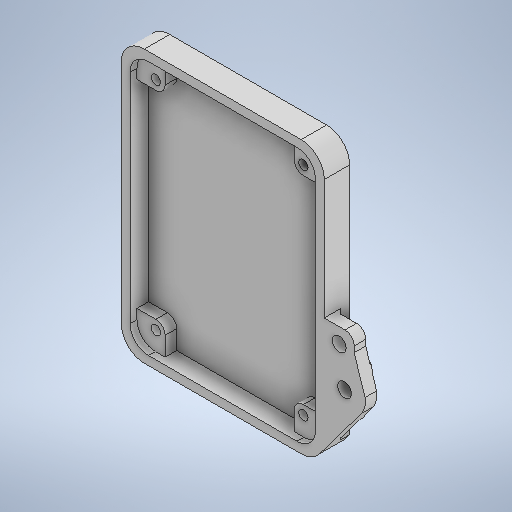
# Autodesk Inventor part: RPi_PD_Trigger
Saved by Autodesk Inventor 2025.1 (Build 291241000, 241)
## iProperties
Created: 2026-04-13
Part Number: RPi_PD_Trigger
Material: Generic
Document SubType Name: Modeling
Designer: User
Density: 1 g/cm^3
Appearance: Default
Author: User
## iProperties of the stored document RPi_PD_Trigger_3DPrint.ipt
Created: 2026-05-05
Part Number: RPi_PD_Trigger_3DPrint
Material: Generic
Document SubType Name: Modeling
Designer: User
Density: 1 g/cm^3
Appearance: Default
Author: User
Autodesk Inventor part; units mm, degrees
ref_plane "YZ Plane" through (0, 0, 0) normal (1, 0, 0) x (0, 1, 0)
ref_plane "XZ Plane" through (0, 0, 0) normal (0, 1, 0) x (-1, 0, 0)
ref_plane "XY Plane" through (0, 0, 0) normal (0, 0, 1) x (1, 0, 0)
sketch "Sketch1" plane through (0, 0, 0) normal (0, 0, 1) x (1, 0, 0)
  line L0 (8.0175, 59.5034) -> (-31.9825, 59.5034)
  line L1 (-31.9825, 59.5034) -> (-31.9825, 4.5034)
  line L2 (-31.9825, 4.5034) -> (8.0175, 4.5034)
  line L3 (8.0175, 4.5034) -> (8.0175, 59.5034)
  line L4 (10.0175, 61.5034) -> (-33.9825, 61.5034)
  line L5 (-33.9825, 61.5034) -> (-33.9825, 2.5034)
  line L6 (-33.9825, 2.5034) -> (10.0175, 2.5034)
  line L7 (10.0175, 2.5034) -> (10.0175, 61.5034)
  line L8 (-32.0825, 4.4034) -> (-32.0825, 59.6034)
  line L9 (-32.0825, 59.6034) -> (8.1175, 59.6034)
  line L10 (8.1175, 59.6034) -> (8.1175, 4.4034)
  line L11 (8.1175, 4.4034) -> (-32.0825, 4.4034)
  point P0 (0, 0)
  dimension "d0" = 40
  dimension "d1" = 55
  dimension "d17" = 2
  dimension "d18" = 59
  dimension "d19" = 44
  dimension "d20" = 0.1
  constraints: 24 end point, 6 parallel, 3 perpendicular, 1 horizontal, 6 other
  measures "d0" distance of L2.end L1.end
  measures "d1" distance of L1.end L0.end
  measures "d17" distance between parallel lines of L3 L7
  measures "d18" distance of L4.end L5.end
  measures "d19" distance of L5.end L6.end
  measures "d20" distance between parallel lines of L1 L8
extrude "Extrusion1" add sketch "Sketch1" along normal blind 5.5 contours L7 L6 L5 L4
sketch "Sketch2" plane through (0, 0, 5.5) normal (0, 0, 1) x (1, 0, 0)
  line L0 (-31.9814, 4.5065) -> (-31.9814, 59.8269) construction
  line L1 (-31.9814, 59.8269) -> (7.0141, 59.8269) construction
  line L2 (7.0141, 59.8269) -> (7.0141, 4.5065) construction
  line L3 (7.0141, 4.5065) -> (-31.9814, 4.5065) construction
  point P0 (0, 0)
  constraints: 2 other
sketch "Sketch5" plane through (0, 0, 0) normal (0, 0, -1) x (-1, 0, 0)
  line L0 (-8.1175, 4.4034) -> (32.0825, 4.4034) projected
  line L1 (-8.1175, 59.6034) -> (-8.1175, 4.4034) projected
  line L2 (32.0825, 4.4034) -> (32.0825, 59.6034) projected
  line L3 (32.0825, 59.6034) -> (-8.1175, 59.6034) projected
  point P0 (0, 0)
extrude "Extrusion4" add sketch "Sketch5" against normal blind 1.5
sketch "Sketch6" plane through (0, 0, 1.5) normal (0, 0, 1) x (1, 0, 0)
  line L0 (10.0175, 61.5034) -> (-33.9825, 61.5034) projected
  line L1 (-33.9825, 61.5034) -> (-33.9825, 2.5034) projected
  line L2 (-33.9825, 2.5034) -> (10.0175, 2.5034) projected
  line L3 (10.0175, 2.5034) -> (10.0175, 61.5034) projected
  line L4 (-33.9825, 61.5034) -> (-25.9825, 61.5034)
  line L5 (-25.9825, 61.5034) -> (-25.9825, 55.5034)
  line L6 (-27.9825, 53.5034) -> (-33.9825, 53.5034)
  line L7 (-33.9825, 53.5034) -> (-33.9825, 61.5034)
  line L8 (10.0175, 61.5034) -> (2.0175, 61.5034)
  line L9 (2.0175, 61.5034) -> (2.0175, 55.5034)
  line L10 (4.0175, 53.5034) -> (10.0175, 53.5034)
  line L11 (10.0175, 53.5034) -> (10.0175, 61.5034)
  line L12 (10.0175, 2.5034) -> (10.0175, 61.5034) projected
  line L13 (10.0175, 2.5034) -> (2.0175, 2.5034)
  line L14 (2.0175, 2.5034) -> (2.0175, 8.5034)
  line L15 (4.0175, 10.5034) -> (10.0175, 10.5034)
  line L16 (10.0175, 10.5034) -> (10.0175, 2.5034)
  line L17 (-33.9825, 2.5034) -> (10.0175, 2.5034) projected
  line L18 (-33.9825, 2.5034) -> (-25.9825, 2.5034)
  line L19 (-25.9825, 2.5034) -> (-25.9825, 8.5034)
  line L20 (-27.9825, 10.5034) -> (-33.9825, 10.5034)
  line L21 (-33.9825, 10.5034) -> (-33.9825, 2.5034)
  arc A0 (-25.9825, 8.5034) -> (-27.9825, 10.5034) centre (-27.9825, 8.5034) ccw
  arc A1 (4.0175, 10.5034) -> (2.0175, 8.5034) centre (4.0175, 8.5034) ccw
  arc A2 (2.0175, 55.5034) -> (4.0175, 53.5034) centre (4.0175, 55.5034) ccw
  arc A3 (-27.9825, 53.5034) -> (-25.9825, 55.5034) centre (-27.9825, 55.5034) ccw
  circle A4 centre (-27.9825, 55.5034) radius 1
  circle A5 centre (4.0175, 55.5034) radius 1
  circle A6 centre (-27.9825, 8.5034) radius 1
  circle A7 centre (4.0175, 8.5034) radius 1
  point P0 (0, 0)
  point P1 (-25.9825, 53.5034)
  point P2 (2.0175, 53.5034)
  point P3 (2.0175, 10.5034)
  point P4 (-25.9825, 10.5034)
  dimension "d24" = 8
  dimension "d25" = 8
  dimension "d26" = 8
  dimension "d27" = 8
  dimension "d28" = 8
  dimension "d29" = 8
  dimension "d30" = 8
  dimension "d31" = 8
  dimension "d32" = 2
  dimension "d33" = 2
  dimension "d34" = 2
  dimension "d35" = 2
  dimension "d36" = 2
  constraints: 32 end point, 8 centre point, 8 parallel, 8 point on circle, 8 point on line, 8 tangent, 4 coincident, 4 horizontal, 4 perpendicular, 3 equal radius
  measures "d24" distance of point (-25.983, 53.503) L6.end
  measures "d25" distance of L4.end point (-25.983, 53.503)
  measures "d26" distance of L10.end point (2.017, 53.503)
  measures "d27" distance of point (2.017, 53.503) L8.end
  measures "d28" distance of point (2.017, 10.503) L15.end
  measures "d29" distance of L13.end point (2.017, 10.503)
  measures "d30" distance of L20.end point (-25.983, 10.503)
  measures "d31" distance of point (-25.983, 10.503) L18.end
  measures "d32" radius of A0
  measures "d33" diameter of A4
  measures "d34" diameter of A5
  measures "d35" diameter of A6
  measures "d36" diameter of A7
extrude "Extrusion5" add sketch "Sketch6" along normal blind 2.5 contours L3 L10 A2 L9 L0 | L5 A3 L6 L1 L0 | L3 L2 L14 A1 L15 | L20 A0 L19 L2 L1
fillet "Fillet2" radius 4 4 edges at (-32.0825, 4.4034, 4.75) (-32.0825, 59.6034, 4.75) (8.1175, 59.6034, 4.75) (8.1175, 4.4034, 4.75)
fillet "Fillet3" radius 5 4 edges at (10.0175, 2.5034, 2.75) (10.0175, 61.5034, 2.75) (-33.9825, 61.5034, 2.75) (-33.9825, 2.5034, 2.75)
sketch "Sketch7" plane through (0, 0, 5.5) normal (0, 0, 1) x (1, 0, 0)
  line L0 (10.0175, 7.5034) -> (10.0175, 56.5034) projected
  line L1 (-28.9825, 2.5034) -> (5.0175, 2.5034) projected
  line L2 (5.0175, 2.5034) -> (5.0175, 30.5034)
  line L3 (10.0175, 30.5034) -> (14.5175, 30.5034)
  line L4 (16.5175, 28.5034) -> (16.5175, 4.5034)
  line L5 (10.0175, 2.5034) -> (10.0175, 30.5034)
  arc A0 (5.0175, 2.5034) -> (10.0175, 7.5034) centre (5.0175, 7.5034) ccw projected
  line L6 (5.0175, 2.5034) -> (14.5175, 2.5034)
  arc A1 (5.0175, 2.5034) -> (10.0175, 7.5034) centre (5.0175, 7.5034) ccw projected
  arc A2 (16.5175, 28.5034) -> (14.5175, 30.5034) centre (14.5175, 28.5034) ccw
  arc A3 (14.5175, 2.5034) -> (16.5175, 4.5034) centre (14.5175, 4.5034) ccw
  line L7 (10.0175, 30.5034) -> (16.5175, 30.5034)
  line L8 (16.5175, 30.5034) -> (16.5175, 24.0034)
  line L9 (16.5175, 24.0034) -> (10.0175, 24.0034)
  line L10 (10.0175, 24.0034) -> (10.0175, 30.5034)
  line L11 (16.5175, 24.0034) -> (10.0175, 30.5034)
  circle A4 centre (13.2675, 27.2534) radius 1.5
  point P0 (0, 0)
  point P1 (16.5175, 2.5034)
  dimension "d42" = 28
  dimension "d44" = 6.5
  dimension "d45" = 2
  dimension "d46" = 2
  dimension "d47" = 6.5
  dimension "d48" = 3
  constraints: 20 end point, 5 tangent, 4 point on circle, 4 point on line, 3 centre point, 3 parallel, 2 horizontal, 2 perpendicular, 1 midpoint, 1 vertical
  measures "d42" distance of L1.end L2.end
  measures "d44" distance of point (16.517, 2.503) L5.start
  measures "d45" radius of A2
  measures "d46" radius of A3
  measures "d47" distance of L7.end L8.end
  measures "d48" diameter of A4
extrude "Extrusion6" add sketch "Sketch7" against normal up to surface (5.5 mm away) contours L0 L9 L4 A3 L6 L5 | L5 L6 A0 | L0 L11 A4 L9 | L3 A2 L4 L11 A4
sketch "Sketch8" plane through (0, 0, 5.5) normal (0, 0, 1) x (1, 0, 0)
  circle A0 centre (14.4423, 19.236) radius 1.5 projected
  point P0 (0, 0)
extrude "Extrusion7" cut sketch "Sketch8" against normal blind 10
sketch "Sketch9" plane through (0, 0, 5.5) normal (0, 0, 1) x (1, 0, 0)
  circle A0 centre (14.4423, 19.236) radius 1.5 projected
  circle A1 centre (14.4423, 19.236) radius 4.5
  line L0 (16.5175, 4.5034) -> (16.5175, 28.5034) projected
  point P0 (0, 0)
  point P1 (16.5175, 23.229)
  point P2 (16.5175, 15.2431)
  dimension "d53" = 3
  constraints: 1 centre point
  measures "d53" radial gap between concentric circles of A0 A1
extrude "Extrusion8" add sketch "Sketch9" against normal up to surface (5.5 mm away) contours A1 L0 picked at (17.8338, 18.9111)
sketch "Sketch10" plane through (0, 0, 5.5) normal (0, 0, 1) x (1, 0, 0)
  line L0 (10.0175, 30.5034) -> (10.0175, 56.5034) projected
  line L1 (-28.9825, 2.5034) -> (14.5175, 2.5034) projected
  line L2 (8.1175, 55.6034) -> (8.1175, 8.4034) projected
  line L3 (4.1175, 4.4034) -> (-28.0825, 4.4034) projected
  line L4 (10.0175, 34.9354) -> (10.0175, 2.5034)
  line L5 (16.5175, 4.5034) -> (16.5175, 15.2431) projected
  line L6 (0, 4.4034) -> (16.5175, 4.5034)
  circle A0 centre (5.0175, 7.5034) radius 5
  arc A1 (16.5175, 15.2431) -> (16.5175, 23.229) centre (14.4423, 19.236) ccw projected
  line L7 (4.2612, -1.838) -> (20.9867, 20.4617)
  arc A2 (14.5175, 2.5034) -> (16.5175, 4.5034) centre (14.5175, 4.5034) ccw projected
  point P0 (0, 0)
  point P1 (16.5175, 14.503)
  point P2 (8.9832, 4.4578)
  point P3 (8.9828, 4.4578)
  point P4 (5.0175, 2.5034)
  dimension "d56" = 10
  constraints: 6 end point, 4 point on line, 4 tangent, 1 centre point
  measures "d56" diameter of A0
extrude "Extrusion9" cut sketch "Sketch10" against normal blind 10 contours L4 L6 A2 L1 | L1 L7 L6 L4 | L1 A0 L7 | L6 L7 L4 | L4 L7 L5 L6
sketch "Sketch11" plane through (0, 0, 5.5) normal (0, 0, 1) x (1, 0, 0)
  arc A0 (16.5175, 15.2431) -> (16.5175, 23.229) centre (14.4423, 19.236) ccw projected
  line L0 (8.9832, 4.4578) -> (16.5175, 14.503) projected
  line L1 (14.193, 11.4039) -> (18.0422, 16.536)
  line L2 (16.5175, 14.503) -> (16.5175, 15.2431) projected
  point P0 (0, 0)
  constraints: 2 end point, 2 point on line, 1 point on circle
extrude "Extrusion10" add sketch "Sketch11" against normal up to surface (5.5 mm away)
chamfer "Chamfer1" distance 4 angle 45 1 edges at (16.5175, 23.229, 2.75)
sketch "Sketch12" plane through (0, 0, 0) normal (0, 0, -1) x (-1, 0, 0)
  line L0 (-10.0175, 30.5034) -> (-10.0175, 56.5034) projected
  line L1 (-10.0175, 30.5034) -> (-14.5175, 30.5034) projected
  arc A0 (-14.5175, 30.5034) -> (-16.5175, 28.5034) centre (-14.5175, 28.5034) ccw projected
  line L2 (-16.5175, 28.5034) -> (-16.5175, 27.229) projected
  line L3 (-18.8771, 19.9991) -> (-16.5175, 27.229) projected
  arc A1 (-18.8771, 19.9991) -> (-18.0422, 16.536) centre (-14.4423, 19.236) ccw projected
  line L4 (-18.0422, 16.536) -> (-8.9832, 4.4578) projected
  arc A2 (-8.9828, 4.4578) -> (-5.0175, 2.5034) centre (-5.0175, 7.5034) ccw projected
  line L5 (-10.0175, 38.8161) -> (-10.0175, 5.8367)
  point P0 (0, 0)
  constraints: 3 point on line, 2 end point
extrude "Extrusion11" cut sketch "Sketch12" against normal blind 3
chamfer "Chamfer2" distance 1 angle 45 1 edges at (10.0175, 18.1701, 3)
sketch "Sketch13" plane through (0, 0, 0) normal (0, 0, -1) x (-1, 0, 0)
  line L0 (-10.0175, 5.8367) -> (-10.0175, 56.5034) projected
  line L1 (-11.0175, 7.17) -> (-18.0422, 16.536) projected
  line L2 (-10.0175, 15.2374) -> (-17.0683, 15.2374)
  line L3 (-10.0175, 15.2374) -> (-10.0175, 12.7374)
  line L4 (-10.0175, 12.7374) -> (-15.1932, 12.7374)
  point P0 (0, 0)
  dimension "d69" = 2.5
  constraints: 6 end point, 4 point on line, 1 horizontal, 1 perpendicular
  measures "d69" distance of L2.start L3.end
extrude "Extrusion12" add sketch "Sketch13" against normal up to surface (3 mm away)
sketch "Sketch14" plane through (10.0175, 12.7374, 0) normal (0, -1, 0) x (1, 0, 0)
  line L0 (7.0508, 0) -> (7.0508, 3) projected
  line L1 (5.1758, 0) -> (0, 0) projected
  line L2 (7.0508, 0) -> (5.1758, 0) projected
  line L3 (0, 2) -> (0, 0) projected
  line L4 (7.0508, 3) -> (0, 0)
  point P0 (-10.0175, 0)
  constraints: 2 end point
extrude "Extrusion13" cut sketch "Sketch14" against normal blind 10
sketch "Sketch15" plane through (0, 0, 0) normal (0, 0, -1) x (-1, 0, 0)
  line L0 (-10.0175, 15.2374) -> (-10.0175, 56.5034) projected
  circle A0 centre (-14.4423, 19.236) radius 1.5 projected
  circle A1 centre (-13.2675, 27.2534) radius 1.5 projected
  line L1 (-10.0175, 19.236) -> (-14.4423, 19.236)
  line L2 (-13.2675, 27.2534) -> (-10.0175, 27.2534)
  line L3 (-18.8771, 19.9991) -> (-16.5175, 27.229) projected
  line L4 (-10.0175, 19.236) -> (-10.0175, 23.236)
  line L5 (-10.0175, 15.2374) -> (-10.0175, 30.5034) projected
  line L6 (-10.0175, 23.236) -> (-17.8207, 23.236)
  line L7 (-17.8207, 24.236) -> (-9.0175, 24.236)
  line L8 (-9.0175, 24.236) -> (-9.0175, 18.236)
  line L9 (-9.0175, 18.236) -> (-14.4423, 18.236)
  line L10 (-17.8207, 22.236) -> (-11.0175, 22.236)
  line L11 (-11.0175, 22.236) -> (-11.0175, 20.236)
  line L12 (-11.0175, 20.236) -> (-14.4423, 20.236)
  line L13 (-18.147, 22.236) -> (-10.0175, 22.236)
  point P0 (0, 0)
  point P1 (-10.0175, 24.236)
  point P2 (-17.4943, 24.236)
  dimension "d74" = 8.0174
  dimension "d75" = 4
  dimension "d76" = 1
  dimension "d77" = 1
  constraints: 22 end point, 7 point on line, 5 perpendicular, 4 other
  measures "d74" distance between parallel lines of L2 L1
  measures "d75" distance of L1.start L4.end
  measures "d76" distance between parallel lines of L6 L7
  measures "d77" distance between parallel lines of L6 L10
extrude "Extrusion14" add sketch "Sketch15" against normal up to surface (3 mm away) contours L13 L10 L3 L6 L0 | L6 L3 L7 L0
sketch "Sketch16" plane through (10.0175, 24.236, 0) normal (0, 1, 0) x (1, 0, 0)
  line L0 (8.1296, 0) -> (8.1296, -3) projected
  line L1 (0, 0) -> (7.4768, 0) projected
  line L2 (7.4768, 0) -> (8.1296, 0) projected
  line L3 (-5, 0) -> (0, 0) projected
  line L4 (8.1296, -3) -> (0, 0)
  point P0 (-10.0175, 0)
  constraints: 2 end point
extrude "Extrusion15" cut sketch "Sketch16" against normal blind 5.25
body "Solid1"
